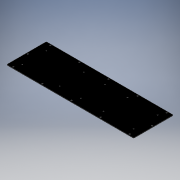
# Autodesk Inventor part: Enclosure2_RevB_Inner
Saved by Autodesk Inventor 2018 (Build 220112000, 112)
## iProperties
Created: 2018-06-27
Part Number: Enclosure2_RevB_Inner
Material: Aluminum 6061
Document SubType Name: Modeling
Designer: Rich
Density: 2.7 g/cm^3
Appearance: Anodized - Black
Author: Rich
Autodesk Inventor part; units mm, degrees
ref_plane "YZ Plane" through (0, 0, 0) normal (1, 0, 0) x (0, 1, 0)
ref_plane "XZ Plane" through (0, 0, 0) normal (0, 1, 0) x (-1, 0, 0)
ref_plane "XY Plane" through (0, 0, 0) normal (0, 0, 1) x (1, 0, 0)
sketch "Sketch4" plane through (0, 0, 0) normal (0, 1, 0) x (-1, 0, 0)
  line L0 (0, -101.6) -> (0, 0)
  line L1 (0, 0) -> (-406.4, 0)
  line L2 (-406.4, 0) -> (-406.4, -101.6)
  line L3 (-406.4, -101.6) -> (0, -101.6)
  circle A0 centre (-397.51, -92.71) radius 1.8986
  circle A1 centre (-292.1, -92.71) radius 1.8986
  circle A2 centre (-213.36, -92.71) radius 1.8986
  circle A3 centre (-139.7, -92.71) radius 1.8986
  circle A4 centre (-8.89, -8.89) radius 1.8986
  circle A5 centre (-381, -92.78) radius 1
  circle A6 centre (-381, -73.73) radius 1
  circle A7 centre (-381, -54.68) radius 1
  circle A8 centre (-381, -35.63) radius 1
  circle A9 centre (-381, -16.58) radius 1
  circle A10 centre (-355.6, -6.28) radius 1
  circle A11 centre (-355.6, -25.33) radius 1
  circle A12 centre (-355.6, -44.38) radius 1
  circle A13 centre (-355.6, -63.43) radius 1
  circle A14 centre (-355.6, -82.48) radius 1
  circle A15 centre (-330.2, -92.78) radius 1
  circle A16 centre (-330.2, -73.73) radius 1
  circle A17 centre (-330.2, -54.68) radius 1
  circle A18 centre (-330.2, -35.63) radius 1
  circle A19 centre (-330.2, -16.58) radius 1
  circle A20 centre (-279.4, -92.78) radius 1
  circle A21 centre (-279.4, -73.73) radius 1
  circle A22 centre (-279.4, -54.68) radius 1
  circle A23 centre (-279.4, -35.63) radius 1
  circle A24 centre (-279.4, -6.28) radius 1
  circle A25 centre (-177.8, -82.48) radius 1
  circle A26 centre (-177.8, -63.43) radius 1
  circle A27 centre (-177.8, -44.38) radius 1
  circle A28 centre (-177.8, -25.33) radius 1
  circle A29 centre (-177.8, -6.28) radius 1
  circle A30 centre (-152.4, -16.58) radius 1
  circle A31 centre (-152.4, -35.63) radius 1
  circle A32 centre (-152.4, -54.68) radius 1
  circle A33 centre (-152.4, -73.73) radius 1
  circle A34 centre (-152.4, -92.78) radius 1
  circle A35 centre (-127, -82.48) radius 1
  circle A36 centre (-127, -63.43) radius 1
  circle A37 centre (-127, -35.63) radius 1
  circle A38 centre (-127, -16.58) radius 1
  circle A39 centre (-76.2, -6.28) radius 1
  circle A40 centre (-76.2, -25.33) radius 1
  circle A41 centre (-76.2, -44.38) radius 1
  circle A42 centre (-76.2, -63.43) radius 1
  circle A43 centre (-76.2, -82.48) radius 1
  circle A44 centre (-382.6, -87.63) radius 0.85
  circle A45 centre (-382.6, -49.53) radius 0.85
  circle A46 centre (-382.6, -11.43) radius 0.85
  circle A47 centre (-357.2, -30.48) radius 0.85
  circle A48 centre (-357.2, -68.58) radius 0.85
  circle A49 centre (-331.8, -87.63) radius 0.85
  circle A50 centre (-331.8, -49.53) radius 0.85
  circle A51 centre (-331.8, -11.43) radius 0.85
  circle A52 centre (-281, -68.58) radius 0.85
  circle A53 centre (-281, -30.48) radius 0.85
  circle A54 centre (-179.4, -87.63) radius 0.85
  circle A55 centre (-179.4, -49.53) radius 0.85
  circle A56 centre (-179.4, -11.43) radius 0.85
  circle A57 centre (-154, -30.48) radius 0.85
  circle A58 centre (-154, -68.58) radius 0.85
  circle A59 centre (-128.6, -87.63) radius 0.85
  circle A60 centre (-128.6, -49.53) radius 0.85
  circle A61 centre (-128.6, -11.43) radius 0.85
  circle A62 centre (-77.8, -30.48) radius 0.85
  circle A63 centre (-77.8, -68.58) radius 0.85
  circle A64 centre (-394.145, -31.5) radius 0.6
  circle A65 centre (-394.145, -38.5) radius 0.6
  circle A66 centre (-394.145, -45.5) radius 0.6
  circle A67 centre (-394.145, -52.5) radius 0.6
  circle A68 centre (-394.145, -59.5) radius 0.6
  circle A69 centre (-394.145, -66.5) radius 0.6
  circle A70 centre (-19.25, -70) radius 0.6
  circle A71 centre (-19.25, -63) radius 0.6
  circle A72 centre (-19.25, -56) radius 0.6
  circle A73 centre (-19.25, -49) radius 0.6
  circle A74 centre (-19.25, -42) radius 0.6
  circle A75 centre (-19.25, -35) radius 0.6
  circle A76 centre (-214.63, -72.39) radius 0.4953
  circle A77 centre (-214.63, -67.31) radius 0.4953
  circle A78 centre (-214.63, -62.23) radius 0.4953
  circle A79 centre (-214.63, -57.15) radius 0.4953
  circle A80 centre (-214.63, -52.07) radius 0.4953
  circle A81 centre (-214.63, -46.99) radius 0.4953
  circle A82 centre (-214.63, -41.91) radius 0.4953
  circle A83 centre (-212.09, -39.37) radius 0.4953
  circle A84 centre (-212.09, -44.45) radius 0.4953
  circle A85 centre (-212.09, -49.53) radius 0.4953
  circle A86 centre (-212.09, -54.61) radius 0.4953
  circle A87 centre (-212.09, -59.69) radius 0.4953
  circle A88 centre (-212.09, -64.77) radius 0.4953
  circle A89 centre (-212.09, -69.85) radius 0.4953
  circle A90 centre (-212.09, -72.39) radius 0.4953
  circle A91 centre (-212.09, -67.31) radius 0.4953
  circle A92 centre (-212.09, -62.23) radius 0.4953
  circle A93 centre (-212.09, -57.15) radius 0.4953
  circle A94 centre (-212.09, -52.07) radius 0.4953
  circle A95 centre (-212.09, -46.99) radius 0.4953
  circle A96 centre (-212.09, -41.91) radius 0.4953
  circle A97 centre (-214.63, -39.37) radius 0.4953
  circle A98 centre (-214.63, -44.45) radius 0.4953
  circle A99 centre (-214.63, -49.53) radius 0.4953
  circle A100 centre (-214.63, -54.61) radius 0.4953
  circle A101 centre (-214.63, -59.69) radius 0.4953
  circle A102 centre (-214.63, -64.77) radius 0.4953
  circle A103 centre (-214.63, -69.85) radius 0.4953
  circle A104 centre (-19.25, -31.5) radius 0.6
  circle A105 centre (-19.25, -38.5) radius 0.6
  circle A106 centre (-19.25, -45.5) radius 0.6
  circle A107 centre (-19.25, -52.5) radius 0.6
  circle A108 centre (-19.25, -59.5) radius 0.6
  circle A109 centre (-19.25, -66.5) radius 0.6
  circle A110 centre (-394.145, -70) radius 0.6
  circle A111 centre (-394.145, -63) radius 0.6
  circle A112 centre (-394.145, -56) radius 0.6
  circle A113 centre (-394.145, -49) radius 0.6
  circle A114 centre (-394.145, -42) radius 0.6
  circle A115 centre (-394.145, -35) radius 0.6
  circle A116 centre (-77.8, -87.63) radius 0.85
  circle A117 centre (-77.8, -49.53) radius 0.85
  circle A118 centre (-77.8, -11.43) radius 0.85
  circle A119 centre (-128.6, -30.48) radius 0.85
  circle A120 centre (-128.6, -68.58) radius 0.85
  circle A121 centre (-154, -87.63) radius 0.85
  circle A122 centre (-154, -49.53) radius 0.85
  circle A123 centre (-154, -11.43) radius 0.85
  circle A124 centre (-179.4, -30.48) radius 0.85
  circle A125 centre (-179.4, -68.58) radius 0.85
  circle A126 centre (-281, -11.43) radius 0.85
  circle A127 centre (-281, -49.53) radius 0.85
  circle A128 centre (-281, -87.63) radius 0.85
  circle A129 centre (-331.8, -30.48) radius 0.85
  circle A130 centre (-331.8, -68.58) radius 0.85
  circle A131 centre (-357.2, -87.63) radius 0.85
  circle A132 centre (-357.2, -49.53) radius 0.85
  circle A133 centre (-357.2, -11.43) radius 0.85
  circle A134 centre (-382.6, -30.48) radius 0.85
  circle A135 centre (-382.6, -68.58) radius 0.85
  circle A136 centre (-76.2, -92.78) radius 1
  circle A137 centre (-76.2, -73.73) radius 1
  circle A138 centre (-76.2, -54.68) radius 1
  circle A139 centre (-76.2, -35.63) radius 1
  circle A140 centre (-76.2, -16.58) radius 1
  circle A141 centre (-127, -6.28) radius 1
  circle A142 centre (-127, -25.33) radius 1
  circle A143 centre (-127, -44.38) radius 1
  circle A144 centre (-127, -73.73) radius 1
  circle A145 centre (-127, -92.78) radius 1
  circle A146 centre (-152.4, -82.48) radius 1
  circle A147 centre (-152.4, -63.43) radius 1
  circle A148 centre (-152.4, -44.38) radius 1
  circle A149 centre (-152.4, -25.33) radius 1
  circle A150 centre (-152.4, -6.28) radius 1
  circle A151 centre (-177.8, -16.58) radius 1
  circle A152 centre (-177.8, -35.63) radius 1
  circle A153 centre (-177.8, -54.68) radius 1
  circle A154 centre (-177.8, -73.73) radius 1
  circle A155 centre (-177.8, -92.78) radius 1
  circle A156 centre (-279.4, -16.58) radius 1
  circle A157 centre (-279.4, -44.38) radius 1
  circle A158 centre (-279.4, -63.43) radius 1
  circle A159 centre (-279.4, -82.48) radius 1
  circle A160 centre (-330.2, -6.28) radius 1
  circle A161 centre (-330.2, -25.33) radius 1
  circle A162 centre (-330.2, -44.38) radius 1
  circle A163 centre (-330.2, -63.43) radius 1
  circle A164 centre (-330.2, -82.48) radius 1
  circle A165 centre (-355.6, -92.78) radius 1
  circle A166 centre (-355.6, -73.73) radius 1
  circle A167 centre (-355.6, -54.68) radius 1
  circle A168 centre (-355.6, -35.63) radius 1
  circle A169 centre (-355.6, -16.58) radius 1
  circle A170 centre (-381, -6.28) radius 1
  circle A171 centre (-381, -25.33) radius 1
  circle A172 centre (-381, -44.38) radius 1
  circle A173 centre (-381, -63.43) radius 1
  circle A174 centre (-381, -82.48) radius 1
  circle A175 centre (-279.4, -25.33) radius 1
  circle A176 centre (-8.89, -92.71) radius 1.8986
  circle A177 centre (-139.7, -8.89) radius 1.8986
  circle A178 centre (-213.36, -8.89) radius 1.8986
  circle A179 centre (-292.1, -8.89) radius 1.8986
  circle A180 centre (-397.51, -8.89) radius 1.8986
  constraints: 181 centre point, 8 end point
sketch "Sketch5" plane through (0, 0, 0) normal (0, 1, 0) x (-1, 0, 0)
  line L0 (-406.4, -101.6) -> (0, -101.6) construction
  line L1 (0, -101.6) -> (0, 0) construction
  line L2 (0, 0) -> (-406.4, 0) construction
  line L3 (-406.4, 0) -> (-406.4, -101.6) construction
  line L4 (-203.2, -101.6) -> (-203.2, 0) construction
  line L5 (0, -50.8) -> (-406.4, -50.8) construction
  line L6 (18.415, -120.015) -> (-424.815, -120.015)
  line L7 (-424.815, -120.015) -> (-424.815, 18.415)
  line L8 (-424.815, 18.415) -> (18.415, 18.415)
  line L9 (18.415, 18.415) -> (18.415, -120.015)
  line L10 (18.415, -120.015) -> (-424.815, 18.415) construction
  line L11 (-424.815, -120.015) -> (18.415, 18.415) construction
  point P0 (-203.2, -50.8)
  dimension "d22" = 443.23
  dimension "d23" = 138.43
  constraints: 16 end point, 7 midpoint, 2 parallel, 1 horizontal, 1 perpendicular
  measures "d22" distance of L6.start L6.end
  measures "d23" distance of L8.end L6.start
extrude "Extrusion3" add sketch "Sketch5" along normal blind 1.5748
sketch "Sketch6" plane through (0, 1.5748, 0) normal (0, 1, 0) x (1, 0, 0)
  circle A0 centre (8.89, 92.71) radius 1.8986 construction
  circle A1 centre (8.89, 8.89) radius 1.8986 construction
  circle A2 centre (139.7, 8.89) radius 1.8986 construction
  circle A3 centre (139.7, 92.71) radius 1.8986 construction
  circle A4 centre (213.36, 92.71) radius 1.8986 construction
  circle A5 centre (213.36, 8.89) radius 1.8986 construction
  circle A6 centre (292.1, 8.89) radius 1.8986 construction
  circle A7 centre (292.1, 92.71) radius 1.8986 construction
  circle A8 centre (397.51, 92.71) radius 1.8986 construction
  circle A9 centre (397.51, 8.89) radius 1.8986 construction
  circle A10 centre (8.89, 8.89) radius 1.7526
  circle A11 centre (8.89, 92.71) radius 1.7526
  circle A12 centre (139.7, 8.89) radius 1.7526
  circle A13 centre (139.7, 92.71) radius 1.7526
  circle A14 centre (213.36, 92.71) radius 1.7526
  circle A15 centre (213.36, 8.89) radius 1.7526
  circle A16 centre (292.1, 8.89) radius 1.8986
  circle A17 centre (292.1, 92.71) radius 1.8986
  circle A18 centre (397.51, 92.71) radius 1.8986
  circle A19 centre (397.51, 8.89) radius 1.8986
  point P0 (0, 0)
  dimension "d26" = 3.5052
  constraints: 10 centre point, 10 coincident, 9 equal radius
  measures "d26" diameter of A10
extrude "Extrusion4" cut sketch "Sketch6" against normal blind 1.5748
sketch "Sketch7" plane through (0, 1.5748, 0) normal (0, 1, 0) x (1, 0, 0)
  line L0 (-18.415, -18.415) -> (-18.415, 120.015) construction
  line L1 (-18.415, 50.8) -> (424.815, 50.8) construction
  line L2 (424.815, 120.015) -> (424.815, -18.415) construction
  line L3 (424.815, -18.415) -> (-18.415, -18.415) construction
  line L4 (203.2, -18.415) -> (203.2, 120.015) construction
  line L5 (-18.415, 120.015) -> (424.815, 120.015) construction
  circle A0 centre (-13.6525, 50.8) radius 1.7526
  circle A1 centre (420.0525, 50.8) radius 1.7526
  circle A2 centre (0, -13.6525) radius 1.7526
  circle A3 centre (101.6, -13.6525) radius 1.7526
  circle A4 centre (203.2, -13.6525) radius 1.7526
  circle A5 centre (304.8, -13.6525) radius 1.7526
  circle A6 centre (406.4, -13.6525) radius 1.7526
  circle A7 centre (0, 115.2525) radius 1.7526
  circle A8 centre (101.6, 115.2525) radius 1.7526
  circle A9 centre (203.2, 115.2525) radius 1.7526
  circle A10 centre (304.8, 115.2525) radius 1.7526
  circle A11 centre (406.4, 115.2525) radius 1.7526
  circle A12 centre (8.89, 8.89) radius 1.7526 projected
  point P0 (0, 0)
  dimension "d31" = 101.6
  dimension "d34" = 128.905
  dimension "d45" = 433.705
  constraints: 12 centre point, 4 end point, 4 midpoint, 2 equal radius, 2 point on line, 1 horizontal, 1 vertical, 21 other
  measures "d31" distance of A2.centre A3.centre
  measures "d34" distance of A2.centre A7.centre
  measures "d45" distance of A0.centre A1.centre
extrude "Extrusion5" cut sketch "Sketch7" against normal blind 1.5748 contours A0 | A1 | A2 | A3 | A4 | A5 | A6 | A7 | A8 | A9 | A10 | A11
chamfer "Chamfer4" distance 0.635 angle 45 12 edges at (-1.7526, 1.5748, 13.6525) (-15.4051, 1.5748, -50.8) (-1.7526, 1.5748, -115.2525) (99.8474, 1.5748, -115.2525) (99.8474, 1.5748, 13.6525) (201.4474, 1.5748, 13.6525) (201.4474, 1.5748, -115.2525) (303.0474, 1.5748, -115.2525) (404.6474, 1.5748, -115.2525) (418.2999, 1.5748, -50.8) (404.6474, 1.5748, 13.6525) (303.0474, 1.5748, 13.6525)
fillet "Fillet1" radius 3.175 4 edges at (424.815, 0.7874, 18.415) (424.815, 0.7874, -120.015) (-18.415, 0.7874, -120.015) (-18.415, 0.7874, 18.415)
body "Solid2"
